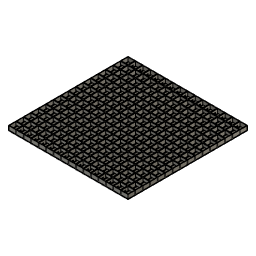
v0_base (Autodesk Fusion 360 design; units mm, degrees)
Autodesk Fusion 360 part; units mm, degrees
(part 1 of 2)
sketch "Skizze5" plane through (0, 0, 0) normal (0, 0, 1) x (1, 0, 0)
  line L0 (0, 272) -> (272, 272)
  line L1 (272, 272) -> (272, 0)
  line L2 (272, 0) -> (0, 0)
  line L3 (0, 0) -> (0, 272)
  dimension "d37" = 272
  dimension "d38" = 272
  constraint horizontal L0
  constraint vertical L1
  constraint horizontal L2
  constraint vertical L3
  constraint coincident L2.end L3.start
  measures "d37" distance of L0.start L0.end
  measures "d38" distance of L0.end L1.end
extrude "Extrusion4" add sketch "Skizze5" along normal blind 10
sketch "Skizze7" plane through (0, 0, 0) normal (0, 0, 1) x (1, 0, 0)
  line L0 (1, 16, 0.0025) -> (16, 16, 0.0025)
  line L1 (16, 16, 0.0025) -> (16, 1, 0.0025)
  line L2 (16, 1, 0.0025) -> (1, 1, 0.0025)
  line L3 (1, 1, 0.0025) -> (1, 16, 0.0025)
  line L4 (18, 16, 0.0025) -> (33, 16, 0.0025)
  line L5 (18, 1, 0.0025) -> (18, 16, 0.0025)
  line L6 (33, 16, 0.0025) -> (33, 1, 0.0025)
  line L7 (33, 1, 0.0025) -> (18, 1, 0.0025)
  line L8 (35, 16, 0.0025) -> (50, 16, 0.0025)
  line L9 (35, 1, 0.0025) -> (35, 16, 0.0025)
  line L10 (50, 16, 0.0025) -> (50, 1, 0.0025)
  line L11 (50, 1, 0.0025) -> (35, 1, 0.0025)
  line L12 (52, 16, 0.0025) -> (67, 16, 0.0025)
  line L13 (52, 1, 0.0025) -> (52, 16, 0.0025)
  line L14 (67, 16, 0.0025) -> (67, 1, 0.0025)
  line L15 (67, 1, 0.0025) -> (52, 1, 0.0025)
  line L16 (69, 16, 0.0025) -> (84, 16, 0.0025)
  line L17 (69, 1, 0.0025) -> (69, 16, 0.0025)
  line L18 (84, 16, 0.0025) -> (84, 1, 0.0025)
  line L19 (84, 1, 0.0025) -> (69, 1, 0.0025)
  line L20 (86, 16, 0.0025) -> (101, 16, 0.0025)
  line L21 (86, 1, 0.0025) -> (86, 16, 0.0025)
  line L22 (101, 16, 0.0025) -> (101, 1, 0.0025)
  line L23 (101, 1, 0.0025) -> (86, 1, 0.0025)
  line L24 (103, 16, 0.0025) -> (118, 16, 0.0025)
  line L25 (103, 1, 0.0025) -> (103, 16, 0.0025)
  line L26 (118, 16, 0.0025) -> (118, 1, 0.0025)
  line L27 (118, 1, 0.0025) -> (103, 1, 0.0025)
  line L28 (120, 16, 0.0025) -> (135, 16, 0.0025)
  line L29 (120, 1, 0.0025) -> (120, 16, 0.0025)
  line L30 (135, 16, 0.0025) -> (135, 1, 0.0025)
  line L31 (135, 1, 0.0025) -> (120, 1, 0.0025)
  line L32 (137, 16, 0.0025) -> (152, 16, 0.0025)
  line L33 (137, 1, 0.0025) -> (137, 16, 0.0025)
  line L34 (152, 16, 0.0025) -> (152, 1, 0.0025)
  line L35 (152, 1, 0.0025) -> (137, 1, 0.0025)
  line L36 (154, 16, 0.0025) -> (169, 16, 0.0025)
  line L37 (154, 1, 0.0025) -> (154, 16, 0.0025)
  line L38 (169, 16, 0.0025) -> (169, 1, 0.0025)
  line L39 (169, 1, 0.0025) -> (154, 1, 0.0025)
  line L40 (171, 16, 0.0025) -> (186, 16, 0.0025)
  line L41 (171, 1, 0.0025) -> (171, 16, 0.0025)
  line L42 (186, 16, 0.0025) -> (186, 1, 0.0025)
  line L43 (186, 1, 0.0025) -> (171, 1, 0.0025)
  line L44 (188, 16, 0.0025) -> (203, 16, 0.0025)
  line L45 (188, 1, 0.0025) -> (188, 16, 0.0025)
  line L46 (203, 16, 0.0025) -> (203, 1, 0.0025)
  line L47 (203, 1, 0.0025) -> (188, 1, 0.0025)
  line L48 (205, 16, 0.0025) -> (220, 16, 0.0025)
  line L49 (205, 1, 0.0025) -> (205, 16, 0.0025)
  line L50 (220, 16, 0.0025) -> (220, 1, 0.0025)
  line L51 (220, 1, 0.0025) -> (205, 1, 0.0025)
  line L52 (222, 16, 0.0025) -> (237, 16, 0.0025)
  line L53 (222, 1, 0.0025) -> (222, 16, 0.0025)
  line L54 (237, 16, 0.0025) -> (237, 1, 0.0025)
  line L55 (237, 1, 0.0025) -> (222, 1, 0.0025)
  line L56 (239, 16, 0.0025) -> (254, 16, 0.0025)
  line L57 (239, 1, 0.0025) -> (239, 16, 0.0025)
  line L58 (254, 16, 0.0025) -> (254, 1, 0.0025)
  line L59 (254, 1, 0.0025) -> (239, 1, 0.0025)
  line L60 (256, 16, 0.0025) -> (271, 16, 0.0025)
  line L61 (256, 1, 0.0025) -> (256, 16, 0.0025)
  line L62 (271, 16, 0.0025) -> (271, 1, 0.0025)
  line L63 (271, 1, 0.0025) -> (256, 1, 0.0025)
  line L64 (1, 33, 0.0025) -> (16, 33, 0.0025)
  line L65 (1, 18, 0.0025) -> (1, 33, 0.0025)
  line L66 (16, 33, 0.0025) -> (16, 18, 0.0025)
  line L67 (16, 18, 0.0025) -> (1, 18, 0.0025)
  line L68 (18, 33, 0.0025) -> (33, 33, 0.0025)
  line L69 (18, 18, 0.0025) -> (18, 33, 0.0025)
  line L70 (33, 33, 0.0025) -> (33, 18, 0.0025)
  line L71 (33, 18, 0.0025) -> (18, 18, 0.0025)
  line L72 (35, 33, 0.0025) -> (50, 33, 0.0025)
  line L73 (35, 18, 0.0025) -> (35, 33, 0.0025)
  line L74 (50, 33, 0.0025) -> (50, 18, 0.0025)
  line L75 (50, 18, 0.0025) -> (35, 18, 0.0025)
  line L76 (52, 33, 0.0025) -> (67, 33, 0.0025)
  line L77 (52, 18, 0.0025) -> (52, 33, 0.0025)
  line L78 (67, 33, 0.0025) -> (67, 18, 0.0025)
  line L79 (67, 18, 0.0025) -> (52, 18, 0.0025)
  line L80 (69, 33, 0.0025) -> (84, 33, 0.0025)
  line L81 (69, 18, 0.0025) -> (69, 33, 0.0025)
  line L82 (84, 33, 0.0025) -> (84, 18, 0.0025)
  line L83 (84, 18, 0.0025) -> (69, 18, 0.0025)
  line L84 (86, 33, 0.0025) -> (101, 33, 0.0025)
  line L85 (86, 18, 0.0025) -> (86, 33, 0.0025)
  line L86 (101, 33, 0.0025) -> (101, 18, 0.0025)
  line L87 (101, 18, 0.0025) -> (86, 18, 0.0025)
  line L88 (103, 33, 0.0025) -> (118, 33, 0.0025)
  line L89 (103, 18, 0.0025) -> (103, 33, 0.0025)
  line L90 (118, 33, 0.0025) -> (118, 18, 0.0025)
  line L91 (118, 18, 0.0025) -> (103, 18, 0.0025)
  line L92 (120, 33, 0.0025) -> (135, 33, 0.0025)
  line L93 (120, 18, 0.0025) -> (120, 33, 0.0025)
  line L94 (135, 33, 0.0025) -> (135, 18, 0.0025)
  line L95 (135, 18, 0.0025) -> (120, 18, 0.0025)
  line L96 (137, 33, 0.0025) -> (152, 33, 0.0025)
  line L97 (137, 18, 0.0025) -> (137, 33, 0.0025)
  line L98 (152, 33, 0.0025) -> (152, 18, 0.0025)
  line L99 (152, 18, 0.0025) -> (137, 18, 0.0025)
  line L100 (154, 33, 0.0025) -> (169, 33, 0.0025)
  line L101 (154, 18, 0.0025) -> (154, 33, 0.0025)
  line L102 (169, 33, 0.0025) -> (169, 18, 0.0025)
  line L103 (169, 18, 0.0025) -> (154, 18, 0.0025)
  line L104 (171, 33, 0.0025) -> (186, 33, 0.0025)
  line L105 (171, 18, 0.0025) -> (171, 33, 0.0025)
  line L106 (186, 33, 0.0025) -> (186, 18, 0.0025)
  line L107 (186, 18, 0.0025) -> (171, 18, 0.0025)
  line L108 (188, 33, 0.0025) -> (203, 33, 0.0025)
  line L109 (188, 18, 0.0025) -> (188, 33, 0.0025)
  line L110 (203, 33, 0.0025) -> (203, 18, 0.0025)
  line L111 (203, 18, 0.0025) -> (188, 18, 0.0025)
  line L112 (205, 33, 0.0025) -> (220, 33, 0.0025)
  line L113 (205, 18, 0.0025) -> (205, 33, 0.0025)
  line L114 (220, 33, 0.0025) -> (220, 18, 0.0025)
  line L115 (220, 18, 0.0025) -> (205, 18, 0.0025)
  line L116 (222, 33, 0.0025) -> (237, 33, 0.0025)
  line L117 (222, 18, 0.0025) -> (222, 33, 0.0025)
  line L118 (237, 33, 0.0025) -> (237, 18, 0.0025)
  line L119 (237, 18, 0.0025) -> (222, 18, 0.0025)
  line L120 (239, 33, 0.0025) -> (254, 33, 0.0025)
  line L121 (239, 18, 0.0025) -> (239, 33, 0.0025)
  line L122 (254, 33, 0.0025) -> (254, 18, 0.0025)
  line L123 (254, 18, 0.0025) -> (239, 18, 0.0025)
  line L124 (256, 33, 0.0025) -> (271, 33, 0.0025)
  line L125 (256, 18, 0.0025) -> (256, 33, 0.0025)
  line L126 (271, 33, 0.0025) -> (271, 18, 0.0025)
  line L127 (271, 18, 0.0025) -> (256, 18, 0.0025)
  line L128 (1, 50, 0.0025) -> (16, 50, 0.0025)
  line L129 (1, 35, 0.0025) -> (1, 50, 0.0025)
  line L130 (16, 50, 0.0025) -> (16, 35, 0.0025)
  line L131 (16, 35, 0.0025) -> (1, 35, 0.0025)
  line L132 (18, 50, 0.0025) -> (33, 50, 0.0025)
  line L133 (18, 35, 0.0025) -> (18, 50, 0.0025)
  line L134 (33, 50, 0.0025) -> (33, 35, 0.0025)
  line L135 (33, 35, 0.0025) -> (18, 35, 0.0025)
  line L136 (35, 50, 0.0025) -> (50, 50, 0.0025)
  line L137 (35, 35, 0.0025) -> (35, 50, 0.0025)
  line L138 (50, 50, 0.0025) -> (50, 35, 0.0025)
  line L139 (50, 35, 0.0025) -> (35, 35, 0.0025)
  line L140 (52, 50, 0.0025) -> (67, 50, 0.0025)
  line L141 (52, 35, 0.0025) -> (52, 50, 0.0025)
  line L142 (67, 50, 0.0025) -> (67, 35, 0.0025)
  line L143 (67, 35, 0.0025) -> (52, 35, 0.0025)
  line L144 (69, 50, 0.0025) -> (84, 50, 0.0025)
  line L145 (69, 35, 0.0025) -> (69, 50, 0.0025)
  line L146 (84, 50, 0.0025) -> (84, 35, 0.0025)
  line L147 (84, 35, 0.0025) -> (69, 35, 0.0025)
  line L148 (86, 50, 0.0025) -> (101, 50, 0.0025)
  line L149 (86, 35, 0.0025) -> (86, 50, 0.0025)
  line L150 (101, 50, 0.0025) -> (101, 35, 0.0025)
  line L151 (101, 35, 0.0025) -> (86, 35, 0.0025)
  line L152 (103, 50, 0.0025) -> (118, 50, 0.0025)
  line L153 (103, 35, 0.0025) -> (103, 50, 0.0025)
  line L154 (118, 50, 0.0025) -> (118, 35, 0.0025)
  line L155 (118, 35, 0.0025) -> (103, 35, 0.0025)
  line L156 (120, 50, 0.0025) -> (135, 50, 0.0025)
  line L157 (120, 35, 0.0025) -> (120, 50, 0.0025)
  line L158 (135, 50, 0.0025) -> (135, 35, 0.0025)
  line L159 (135, 35, 0.0025) -> (120, 35, 0.0025)
  line L160 (137, 50, 0.0025) -> (152, 50, 0.0025)
  line L161 (137, 35, 0.0025) -> (137, 50, 0.0025)
  line L162 (152, 50, 0.0025) -> (152, 35, 0.0025)
  line L163 (152, 35, 0.0025) -> (137, 35, 0.0025)
  line L164 (154, 50, 0.0025) -> (169, 50, 0.0025)
  line L165 (154, 35, 0.0025) -> (154, 50, 0.0025)
  line L166 (169, 50, 0.0025) -> (169, 35, 0.0025)
  line L167 (169, 35, 0.0025) -> (154, 35, 0.0025)
  line L168 (171, 50, 0.0025) -> (186, 50, 0.0025)
  line L169 (171, 35, 0.0025) -> (171, 50, 0.0025)
  line L170 (186, 50, 0.0025) -> (186, 35, 0.0025)
  line L171 (186, 35, 0.0025) -> (171, 35, 0.0025)
  line L172 (188, 50, 0.0025) -> (203, 50, 0.0025)
  line L173 (188, 35, 0.0025) -> (188, 50, 0.0025)
  line L174 (203, 50, 0.0025) -> (203, 35, 0.0025)
  line L175 (203, 35, 0.0025) -> (188, 35, 0.0025)
  line L176 (205, 50, 0.0025) -> (220, 50, 0.0025)
  line L177 (205, 35, 0.0025) -> (205, 50, 0.0025)
  line L178 (220, 50, 0.0025) -> (220, 35, 0.0025)
  line L179 (220, 35, 0.0025) -> (205, 35, 0.0025)
  line L180 (222, 50, 0.0025) -> (237, 50, 0.0025)
  line L181 (222, 35, 0.0025) -> (222, 50, 0.0025)
  line L182 (237, 50, 0.0025) -> (237, 35, 0.0025)
  line L183 (237, 35, 0.0025) -> (222, 35, 0.0025)
  line L184 (239, 50, 0.0025) -> (254, 50, 0.0025)
  line L185 (239, 35, 0.0025) -> (239, 50, 0.0025)
  line L186 (254, 50, 0.0025) -> (254, 35, 0.0025)
  line L187 (254, 35, 0.0025) -> (239, 35, 0.0025)
  line L188 (256, 50, 0.0025) -> (271, 50, 0.0025)
  line L189 (256, 35, 0.0025) -> (256, 50, 0.0025)
  line L190 (271, 50, 0.0025) -> (271, 35, 0.0025)
  line L191 (271, 35, 0.0025) -> (256, 35, 0.0025)
  line L192 (1, 67, 0.0025) -> (16, 67, 0.0025)
  line L193 (1, 52, 0.0025) -> (1, 67, 0.0025)
  line L194 (16, 67, 0.0025) -> (16, 52, 0.0025)
  line L195 (16, 52, 0.0025) -> (1, 52, 0.0025)
  line L196 (18, 67, 0.0025) -> (33, 67, 0.0025)
  line L197 (18, 52, 0.0025) -> (18, 67, 0.0025)
  line L198 (33, 67, 0.0025) -> (33, 52, 0.0025)
  line L199 (33, 52, 0.0025) -> (18, 52, 0.0025)
  line L200 (35, 67, 0.0025) -> (50, 67, 0.0025)
  line L201 (35, 52, 0.0025) -> (35, 67, 0.0025)
  line L202 (50, 67, 0.0025) -> (50, 52, 0.0025)
  line L203 (50, 52, 0.0025) -> (35, 52, 0.0025)
  line L204 (52, 67, 0.0025) -> (67, 67, 0.0025)
  line L205 (52, 52, 0.0025) -> (52, 67, 0.0025)
  line L206 (67, 67, 0.0025) -> (67, 52, 0.0025)
  line L207 (67, 52, 0.0025) -> (52, 52, 0.0025)
  line L208 (69, 67, 0.0025) -> (84, 67, 0.0025)
  line L209 (69, 52, 0.0025) -> (69, 67, 0.0025)
  line L210 (84, 67, 0.0025) -> (84, 52, 0.0025)
  line L211 (84, 52, 0.0025) -> (69, 52, 0.0025)
  line L212 (86, 67, 0.0025) -> (101, 67, 0.0025)
  line L213 (86, 52, 0.0025) -> (86, 67, 0.0025)
  line L214 (101, 67, 0.0025) -> (101, 52, 0.0025)
  line L215 (101, 52, 0.0025) -> (86, 52, 0.0025)
  line L216 (103, 67, 0.0025) -> (118, 67, 0.0025)
  line L217 (103, 52, 0.0025) -> (103, 67, 0.0025)
  line L218 (118, 67, 0.0025) -> (118, 52, 0.0025)
  line L219 (118, 52, 0.0025) -> (103, 52, 0.0025)
  line L220 (120, 67, 0.0025) -> (135, 67, 0.0025)
  line L221 (120, 52, 0.0025) -> (120, 67, 0.0025)
  line L222 (135, 67, 0.0025) -> (135, 52, 0.0025)
  line L223 (135, 52, 0.0025) -> (120, 52, 0.0025)
  line L224 (137, 67, 0.0025) -> (152, 67, 0.0025)
  line L225 (137, 52, 0.0025) -> (137, 67, 0.0025)
  line L226 (152, 67, 0.0025) -> (152, 52, 0.0025)
  line L227 (152, 52, 0.0025) -> (137, 52, 0.0025)
  line L228 (154, 67, 0.0025) -> (169, 67, 0.0025)
  line L229 (154, 52, 0.0025) -> (154, 67, 0.0025)
  line L230 (169, 67, 0.0025) -> (169, 52, 0.0025)
  line L231 (169, 52, 0.0025) -> (154, 52, 0.0025)
  line L232 (171, 67, 0.0025) -> (186, 67, 0.0025)
  line L233 (171, 52, 0.0025) -> (171, 67, 0.0025)
  line L234 (186, 67, 0.0025) -> (186, 52, 0.0025)
  line L235 (186, 52, 0.0025) -> (171, 52, 0.0025)
  line L236 (188, 67, 0.0025) -> (203, 67, 0.0025)
  line L237 (188, 52, 0.0025) -> (188, 67, 0.0025)
  line L238 (203, 67, 0.0025) -> (203, 52, 0.0025)
  line L239 (203, 52, 0.0025) -> (188, 52, 0.0025)
  line L240 (205, 67, 0.0025) -> (220, 67, 0.0025)
  line L241 (205, 52, 0.0025) -> (205, 67, 0.0025)
  line L242 (220, 67, 0.0025) -> (220, 52, 0.0025)
  line L243 (220, 52, 0.0025) -> (205, 52, 0.0025)
  line L244 (222, 67, 0.0025) -> (237, 67, 0.0025)
  line L245 (222, 52, 0.0025) -> (222, 67, 0.0025)
  line L246 (237, 67, 0.0025) -> (237, 52, 0.0025)
  line L247 (237, 52, 0.0025) -> (222, 52, 0.0025)
  line L248 (239, 67, 0.0025) -> (254, 67, 0.0025)
  line L249 (239, 52, 0.0025) -> (239, 67, 0.0025)
  line L250 (254, 67, 0.0025) -> (254, 52, 0.0025)
  line L251 (254, 52, 0.0025) -> (239, 52, 0.0025)
  line L252 (256, 67, 0.0025) -> (271, 67, 0.0025)
  line L253 (256, 52, 0.0025) -> (256, 67, 0.0025)
  line L254 (271, 67, 0.0025) -> (271, 52, 0.0025)
  line L255 (271, 52, 0.0025) -> (256, 52, 0.0025)
  line L256 (1, 84, 0.0025) -> (16, 84, 0.0025)
  line L257 (1, 69, 0.0025) -> (1, 84, 0.0025)
  line L258 (16, 84, 0.0025) -> (16, 69, 0.0025)
  line L259 (16, 69, 0.0025) -> (1, 69, 0.0025)
  line L260 (18, 84, 0.0025) -> (33, 84, 0.0025)
  line L261 (18, 69, 0.0025) -> (18, 84, 0.0025)
  line L262 (33, 84, 0.0025) -> (33, 69, 0.0025)
  line L263 (33, 69, 0.0025) -> (18, 69, 0.0025)
  line L264 (35, 84, 0.0025) -> (50, 84, 0.0025)
  line L265 (35, 69, 0.0025) -> (35, 84, 0.0025)
  line L266 (50, 84, 0.0025) -> (50, 69, 0.0025)
  line L267 (50, 69, 0.0025) -> (35, 69, 0.0025)
  line L268 (52, 84, 0.0025) -> (67, 84, 0.0025)
  line L269 (52, 69, 0.0025) -> (52, 84, 0.0025)
  line L270 (67, 84, 0.0025) -> (67, 69, 0.0025)
  line L271 (67, 69, 0.0025) -> (52, 69, 0.0025)
  line L272 (69, 84, 0.0025) -> (84, 84, 0.0025)
  line L273 (69, 69, 0.0025) -> (69, 84, 0.0025)
  line L274 (84, 84, 0.0025) -> (84, 69, 0.0025)
  line L275 (84, 69, 0.0025) -> (69, 69, 0.0025)
  line L276 (86, 84, 0.0025) -> (101, 84, 0.0025)
  line L277 (86, 69, 0.0025) -> (86, 84, 0.0025)
  line L278 (101, 84, 0.0025) -> (101, 69, 0.0025)
  line L279 (101, 69, 0.0025) -> (86, 69, 0.0025)
  line L280 (103, 84, 0.0025) -> (118, 84, 0.0025)
  line L281 (103, 69, 0.0025) -> (103, 84, 0.0025)
  line L282 (118, 84, 0.0025) -> (118, 69, 0.0025)
  line L283 (118, 69, 0.0025) -> (103, 69, 0.0025)
  line L284 (120, 84, 0.0025) -> (135, 84, 0.0025)
  line L285 (120, 69, 0.0025) -> (120, 84, 0.0025)
  line L286 (135, 84, 0.0025) -> (135, 69, 0.0025)
  line L287 (135, 69, 0.0025) -> (120, 69, 0.0025)
  line L288 (137, 84, 0.0025) -> (152, 84, 0.0025)
  line L289 (137, 69, 0.0025) -> (137, 84, 0.0025)
  line L290 (152, 84, 0.0025) -> (152, 69, 0.0025)
  line L291 (152, 69, 0.0025) -> (137, 69, 0.0025)
  line L292 (154, 84, 0.0025) -> (169, 84, 0.0025)
  line L293 (154, 69, 0.0025) -> (154, 84, 0.0025)
  line L294 (169, 84, 0.0025) -> (169, 69, 0.0025)
  line L295 (169, 69, 0.0025) -> (154, 69, 0.0025)
  line L296 (171, 84, 0.0025) -> (186, 84, 0.0025)
  line L297 (171, 69, 0.0025) -> (171, 84, 0.0025)
  line L298 (186, 84, 0.0025) -> (186, 69, 0.0025)
  line L299 (186, 69, 0.0025) -> (171, 69, 0.0025)
  line L300 (188, 84, 0.0025) -> (203, 84, 0.0025)
  line L301 (188, 69, 0.0025) -> (188, 84, 0.0025)
  line L302 (203, 84, 0.0025) -> (203, 69, 0.0025)
  line L303 (203, 69, 0.0025) -> (188, 69, 0.0025)
  line L304 (205, 84, 0.0025) -> (220, 84, 0.0025)
  line L305 (205, 69, 0.0025) -> (205, 84, 0.0025)
  line L306 (220, 84, 0.0025) -> (220, 69, 0.0025)
  line L307 (220, 69, 0.0025) -> (205, 69, 0.0025)
  line L308 (222, 84, 0.0025) -> (237, 84, 0.0025)
  line L309 (222, 69, 0.0025) -> (222, 84, 0.0025)
  line L310 (237, 84, 0.0025) -> (237, 69, 0.0025)
  line L311 (237, 69, 0.0025) -> (222, 69, 0.0025)
  line L312 (239, 84, 0.0025) -> (254, 84, 0.0025)
  line L313 (239, 69, 0.0025) -> (239, 84, 0.0025)
  line L314 (254, 84, 0.0025) -> (254, 69, 0.0025)
  line L315 (254, 69, 0.0025) -> (239, 69, 0.0025)
  line L316 (256, 84, 0.0025) -> (271, 84, 0.0025)
  line L317 (256, 69, 0.0025) -> (256, 84, 0.0025)
  line L318 (271, 84, 0.0025) -> (271, 69, 0.0025)
  line L319 (271, 69, 0.0025) -> (256, 69, 0.0025)
  line L320 (1, 101, 0.0025) -> (16, 101, 0.0025)
  line L321 (1, 86, 0.0025) -> (1, 101, 0.0025)
  line L322 (16, 101, 0.0025) -> (16, 86, 0.0025)
  line L323 (16, 86, 0.0025) -> (1, 86, 0.0025)
  line L324 (18, 101, 0.0025) -> (33, 101, 0.0025)
  line L325 (18, 86, 0.0025) -> (18, 101, 0.0025)
  line L326 (33, 101, 0.0025) -> (33, 86, 0.0025)
  line L327 (33, 86, 0.0025) -> (18, 86, 0.0025)
  line L328 (35, 101, 0.0025) -> (50, 101, 0.0025)
  line L329 (35, 86, 0.0025) -> (35, 101, 0.0025)
  line L330 (50, 101, 0.0025) -> (50, 86, 0.0025)
  line L331 (50, 86, 0.0025) -> (35, 86, 0.0025)
  line L332 (52, 101, 0.0025) -> (67, 101, 0.0025)
  line L333 (52, 86, 0.0025) -> (52, 101, 0.0025)
  line L334 (67, 101, 0.0025) -> (67, 86, 0.0025)
  line L335 (67, 86, 0.0025) -> (52, 86, 0.0025)
  line L336 (69, 101, 0.0025) -> (84, 101, 0.0025)
  line L337 (69, 86, 0.0025) -> (69, 101, 0.0025)
  line L338 (84, 101, 0.0025) -> (84, 86, 0.0025)
  line L339 (84, 86, 0.0025) -> (69, 86, 0.0025)
  line L340 (86, 101, 0.0025) -> (101, 101, 0.0025)
  line L341 (86, 86, 0.0025) -> (86, 101, 0.0025)
  line L342 (101, 101, 0.0025) -> (101, 86, 0.0025)
  line L343 (101, 86, 0.0025) -> (86, 86, 0.0025)
  line L344 (103, 101, 0.0025) -> (118, 101, 0.0025)
  line L345 (103, 86, 0.0025) -> (103, 101, 0.0025)
  line L346 (118, 101, 0.0025) -> (118, 86, 0.0025)
  line L347 (118, 86, 0.0025) -> (103, 86, 0.0025)
  line L348 (120, 101, 0.0025) -> (135, 101, 0.0025)
  line L349 (120, 86, 0.0025) -> (120, 101, 0.0025)
  line L350 (135, 101, 0.0025) -> (135, 86, 0.0025)
  line L351 (135, 86, 0.0025) -> (120, 86, 0.0025)
  line L352 (137, 101, 0.0025) -> (152, 101, 0.0025)
  line L353 (137, 86, 0.0025) -> (137, 101, 0.0025)
  line L354 (152, 101, 0.0025) -> (152, 86, 0.0025)
  line L355 (152, 86, 0.0025) -> (137, 86, 0.0025)
  line L356 (154, 101, 0.0025) -> (169, 101, 0.0025)
  line L357 (154, 86, 0.0025) -> (154, 101, 0.0025)
  line L358 (169, 101, 0.0025) -> (169, 86, 0.0025)
  line L359 (169, 86, 0.0025) -> (154, 86, 0.0025)
  line L360 (171, 101, 0.0025) -> (186, 101, 0.0025)
  line L361 (171, 86, 0.0025) -> (171, 101, 0.0025)
  line L362 (186, 101, 0.0025) -> (186, 86, 0.0025)
  line L363 (186, 86, 0.0025) -> (171, 86, 0.0025)
  line L364 (188, 101, 0.0025) -> (203, 101, 0.0025)
  line L365 (188, 86, 0.0025) -> (188, 101, 0.0025)
  line L366 (203, 101, 0.0025) -> (203, 86, 0.0025)
  line L367 (203, 86, 0.0025) -> (188, 86, 0.0025)
  line L368 (205, 101, 0.0025) -> (220, 101, 0.0025)
  line L369 (205, 86, 0.0025) -> (205, 101, 0.0025)
  line L370 (220, 101, 0.0025) -> (220, 86, 0.0025)
  line L371 (220, 86, 0.0025) -> (205, 86, 0.0025)
  line L372 (222, 101, 0.0025) -> (237, 101, 0.0025)
  line L373 (222, 86, 0.0025) -> (222, 101, 0.0025)
  line L374 (237, 101, 0.0025) -> (237, 86, 0.0025)
  line L375 (237, 86, 0.0025) -> (222, 86, 0.0025)
  line L376 (239, 101, 0.0025) -> (254, 101, 0.0025)
  line L377 (239, 86, 0.0025) -> (239, 101, 0.0025)
  line L378 (254, 101, 0.0025) -> (254, 86, 0.0025)
  line L379 (254, 86, 0.0025) -> (239, 86, 0.0025)
  line L380 (256, 101, 0.0025) -> (271, 101, 0.0025)
  line L381 (256, 86, 0.0025) -> (256, 101, 0.0025)
  line L382 (271, 101, 0.0025) -> (271, 86, 0.0025)
  line L383 (271, 86, 0.0025) -> (256, 86, 0.0025)
  line L384 (1, 118, 0.0025) -> (16, 118, 0.0025)
  line L385 (1, 103, 0.0025) -> (1, 118, 0.0025)
  line L386 (16, 118, 0.0025) -> (16, 103, 0.0025)
  line L387 (16, 103, 0.0025) -> (1, 103, 0.0025)
  line L388 (18, 118, 0.0025) -> (33, 118, 0.0025)
  line L389 (18, 103, 0.0025) -> (18, 118, 0.0025)
  line L390 (33, 118, 0.0025) -> (33, 103, 0.0025)
  line L391 (33, 103, 0.0025) -> (18, 103, 0.0025)
  line L392 (35, 118, 0.0025) -> (50, 118, 0.0025)
  line L393 (35, 103, 0.0025) -> (35, 118, 0.0025)
  line L394 (50, 118, 0.0025) -> (50, 103, 0.0025)
  line L395 (50, 103, 0.0025) -> (35, 103, 0.0025)
  line L396 (52, 118, 0.0025) -> (67, 118, 0.0025)
  line L397 (52, 103, 0.0025) -> (52, 118, 0.0025)
  line L398 (67, 118, 0.0025) -> (67, 103, 0.0025)
  line L399 (67, 103, 0.0025) -> (52, 103, 0.0025)
  line L400 (69, 118, 0.0025) -> (84, 118, 0.0025)
  line L401 (69, 103, 0.0025) -> (69, 118, 0.0025)
  line L402 (84, 118, 0.0025) -> (84, 103, 0.0025)
  line L403 (84, 103, 0.0025) -> (69, 103, 0.0025)
  line L404 (86, 118, 0.0025) -> (101, 118, 0.0025)
  line L405 (86, 103, 0.0025) -> (86, 118, 0.0025)
  line L406 (101, 118, 0.0025) -> (101, 103, 0.0025)
  line L407 (101, 103, 0.0025) -> (86, 103, 0.0025)
  line L408 (103, 118, 0.0025) -> (118, 118, 0.0025)
  line L409 (103, 103, 0.0025) -> (103, 118, 0.0025)
  line L410 (118, 118, 0.0025) -> (118, 103, 0.0025)
  line L411 (118, 103, 0.0025) -> (103, 103, 0.0025)
  line L412 (120, 118, 0.0025) -> (135, 118, 0.0025)
  line L413 (120, 103, 0.0025) -> (120, 118, 0.0025)
  line L414 (135, 118, 0.0025) -> (135, 103, 0.0025)
  line L415 (135, 103, 0.0025) -> (120, 103, 0.0025)
  line L416 (137, 118, 0.0025) -> (152, 118, 0.0025)
  line L417 (137, 103, 0.0025) -> (137, 118, 0.0025)
  line L418 (152, 118, 0.0025) -> (152, 103, 0.0025)
  line L419 (152, 103, 0.0025) -> (137, 103, 0.0025)
  line L420 (154, 118, 0.0025) -> (169, 118, 0.0025)
  line L421 (154, 103, 0.0025) -> (154, 118, 0.0025)
  line L422 (169, 118, 0.0025) -> (169, 103, 0.0025)
  line L423 (169, 103, 0.0025) -> (154, 103, 0.0025)
  line L424 (171, 118, 0.0025) -> (186, 118, 0.0025)
  line L425 (171, 103, 0.0025) -> (171, 118, 0.0025)
  line L426 (186, 118, 0.0025) -> (186, 103, 0.0025)
  line L427 (186, 103, 0.0025) -> (171, 103, 0.0025)
  line L428 (188, 118, 0.0025) -> (203, 118, 0.0025)
  line L429 (188, 103, 0.0025) -> (188, 118, 0.0025)
  line L430 (203, 118, 0.0025) -> (203, 103, 0.0025)
  line L431 (203, 103, 0.0025) -> (188, 103, 0.0025)
  line L432 (205, 118, 0.0025) -> (220, 118, 0.0025)
  line L433 (205, 103, 0.0025) -> (205, 118, 0.0025)
  line L434 (220, 118, 0.0025) -> (220, 103, 0.0025)
  line L435 (220, 103, 0.0025) -> (205, 103, 0.0025)
  line L436 (222, 118, 0.0025) -> (237, 118, 0.0025)
  line L437 (222, 103, 0.0025) -> (222, 118, 0.0025)
  line L438 (237, 118, 0.0025) -> (237, 103, 0.0025)
  line L439 (237, 103, 0.0025) -> (222, 103, 0.0025)
  line L440 (239, 118, 0.0025) -> (254, 118, 0.0025)
  line L441 (239, 103, 0.0025) -> (239, 118, 0.0025)
  line L442 (254, 118, 0.0025) -> (254, 103, 0.0025)
  line L443 (254, 103, 0.0025) -> (239, 103, 0.0025)
  line L444 (256, 118, 0.0025) -> (271, 118, 0.0025)
  line L445 (256, 103, 0.0025) -> (256, 118, 0.0025)
  line L446 (271, 118, 0.0025) -> (271, 103, 0.0025)
  line L447 (271, 103, 0.0025) -> (256, 103, 0.0025)
  line L448 (1, 135, 0.0025) -> (16, 135, 0.0025)
  line L449 (1, 120, 0.0025) -> (1, 135, 0.0025)
  line L450 (16, 135, 0.0025) -> (16, 120, 0.0025)
  line L451 (16, 120, 0.0025) -> (1, 120, 0.0025)
  line L452 (18, 135, 0.0025) -> (33, 135, 0.0025)
  line L453 (18, 120, 0.0025) -> (18, 135, 0.0025)
  line L454 (33, 135, 0.0025) -> (33, 120, 0.0025)
  line L455 (33, 120, 0.0025) -> (18, 120, 0.0025)
  line L456 (35, 135, 0.0025) -> (50, 135, 0.0025)
  line L457 (35, 120, 0.0025) -> (35, 135, 0.0025)
  line L458 (50, 135, 0.0025) -> (50, 120, 0.0025)
  line L459 (50, 120, 0.0025) -> (35, 120, 0.0025)
  line L460 (52, 135, 0.0025) -> (67, 135, 0.0025)
  line L461 (52, 120, 0.0025) -> (52, 135, 0.0025)
  line L462 (67, 135, 0.0025) -> (67, 120, 0.0025)
  line L463 (67, 120, 0.0025) -> (52, 120, 0.0025)
  line L464 (69, 135, 0.0025) -> (84, 135, 0.0025)
  line L465 (69, 120, 0.0025) -> (69, 135, 0.0025)
  line L466 (84, 135, 0.0025) -> (84, 120, 0.0025)
  line L467 (84, 120, 0.0025) -> (69, 120, 0.0025)
  line L468 (86, 135, 0.0025) -> (101, 135, 0.0025)
  line L469 (86, 120, 0.0025) -> (86, 135, 0.0025)
  line L470 (101, 135, 0.0025) -> (101, 120, 0.0025)
  line L471 (101, 120, 0.0025) -> (86, 120, 0.0025)
  line L472 (103, 135, 0.0025) -> (118, 135, 0.0025)
  line L473 (103, 120, 0.0025) -> (103, 135, 0.0025)
  line L474 (118, 135, 0.0025) -> (118, 120, 0.0025)
  line L475 (118, 120, 0.0025) -> (103, 120, 0.0025)
  line L476 (120, 135, 0.0025) -> (135, 135, 0.0025)
  line L477 (120, 120, 0.0025) -> (120, 135, 0.0025)
  line L478 (135, 135, 0.0025) -> (135, 120, 0.0025)
  line L479 (135, 120, 0.0025) -> (120, 120, 0.0025)
  line L480 (137, 135, 0.0025) -> (152, 135, 0.0025)
  line L481 (137, 120, 0.0025) -> (137, 135, 0.0025)
  line L482 (152, 135, 0.0025) -> (152, 120, 0.0025)
  line L483 (152, 120, 0.0025) -> (137, 120, 0.0025)
  line L484 (154, 135, 0.0025) -> (169, 135, 0.0025)
  line L485 (154, 120, 0.0025) -> (154, 135, 0.0025)
  line L486 (169, 135, 0.0025) -> (169, 120, 0.0025)
  line L487 (169, 120, 0.0025) -> (154, 120, 0.0025)
  line L488 (171, 135, 0.0025) -> (186, 135, 0.0025)
  line L489 (171, 120, 0.0025) -> (171, 135, 0.0025)
  line L490 (186, 135, 0.0025) -> (186, 120, 0.0025)
  line L491 (186, 120, 0.0025) -> (171, 120, 0.0025)
  line L492 (188, 135, 0.0025) -> (203, 135, 0.0025)
  line L493 (188, 120, 0.0025) -> (188, 135, 0.0025)
  line L494 (203, 135, 0.0025) -> (203, 120, 0.0025)
  line L495 (203, 120, 0.0025) -> (188, 120, 0.0025)
  line L496 (205, 135, 0.0025) -> (220, 135, 0.0025)
  line L497 (205, 120, 0.0025) -> (205, 135, 0.0025)
  line L498 (220, 135, 0.0025) -> (220, 120, 0.0025)
  line L499 (220, 120, 0.0025) -> (205, 120, 0.0025)
  line L500 (222, 135, 0.0025) -> (237, 135, 0.0025)
  line L501 (222, 120, 0.0025) -> (222, 135, 0.0025)
  line L502 (237, 135, 0.0025) -> (237, 120, 0.0025)
  line L503 (237, 120, 0.0025) -> (222, 120, 0.0025)
  line L504 (239, 135, 0.0025) -> (254, 135, 0.0025)
  line L505 (239, 120, 0.0025) -> (239, 135, 0.0025)
  line L506 (254, 135, 0.0025) -> (254, 120, 0.0025)
  line L507 (254, 120, 0.0025) -> (239, 120, 0.0025)
  line L508 (256, 135, 0.0025) -> (271, 135, 0.0025)
  line L509 (256, 120, 0.0025) -> (256, 135, 0.0025)
  line L510 (271, 135, 0.0025) -> (271, 120, 0.0025)
  line L511 (271, 120, 0.0025) -> (256, 120, 0.0025)
  line L512 (1, 152, 0.0025) -> (16, 152, 0.0025)
  line L513 (1, 137, 0.0025) -> (1, 152, 0.0025)
  line L514 (16, 152, 0.0025) -> (16, 137, 0.0025)
  line L515 (16, 137, 0.0025) -> (1, 137, 0.0025)
  line L516 (18, 152, 0.0025) -> (33, 152, 0.0025)
  line L517 (18, 137, 0.0025) -> (18, 152, 0.0025)
  line L518 (33, 152, 0.0025) -> (33, 137, 0.0025)
  line L519 (33, 137, 0.0025) -> (18, 137, 0.0025)
  line L520 (35, 152, 0.0025) -> (50, 152, 0.0025)
  line L521 (35, 137, 0.0025) -> (35, 152, 0.0025)
  line L522 (50, 152, 0.0025) -> (50, 137, 0.0025)
  line L523 (50, 137, 0.0025) -> (35, 137, 0.0025)
  line L524 (52, 152, 0.0025) -> (67, 152, 0.0025)
  line L525 (52, 137, 0.0025) -> (52, 152, 0.0025)
  line L526 (67, 152, 0.0025) -> (67, 137, 0.0025)
  line L527 (67, 137, 0.0025) -> (52, 137, 0.0025)
  line L528 (69, 152, 0.0025) -> (84, 152, 0.0025)
  line L529 (69, 137, 0.0025) -> (69, 152, 0.0025)
  line L530 (84, 152, 0.0025) -> (84, 137, 0.0025)
  line L531 (84, 137, 0.0025) -> (69, 137, 0.0025)
  line L532 (86, 152, 0.0025) -> (101, 152, 0.0025)
  line L533 (86, 137, 0.0025) -> (86, 152, 0.0025)
  line L534 (101, 152, 0.0025) -> (101, 137, 0.0025)
  line L535 (101, 137, 0.0025) -> (86, 137, 0.0025)
  line L536 (103, 152, 0.0025) -> (118, 152, 0.0025)
  line L537 (103, 137, 0.0025) -> (103, 152, 0.0025)
  line L538 (118, 152, 0.0025) -> (118, 137, 0.0025)
  line L539 (118, 137, 0.0025) -> (103, 137, 0.0025)
  line L540 (120, 152, 0.0025) -> (135, 152, 0.0025)
  line L541 (120, 137, 0.0025) -> (120, 152, 0.0025)
  line L542 (135, 152, 0.0025) -> (135, 137, 0.0025)
  line L543 (135, 137, 0.0025) -> (120, 137, 0.0025)
  line L544 (137, 152, 0.0025) -> (152, 152, 0.0025)
  line L545 (137, 137, 0.0025) -> (137, 152, 0.0025)
  line L546 (152, 152, 0.0025) -> (152, 137, 0.0025)
  line L547 (152, 137, 0.0025) -> (137, 137, 0.0025)
  line L548 (154, 152, 0.0025) -> (169, 152, 0.0025)
  line L549 (154, 137, 0.0025) -> (154, 152, 0.0025)
  line L550 (169, 152, 0.0025) -> (169, 137, 0.0025)
  line L551 (169, 137, 0.0025) -> (154, 137, 0.0025)
  line L552 (171, 152, 0.0025) -> (186, 152, 0.0025)
  line L553 (171, 137, 0.0025) -> (171, 152, 0.0025)
  line L554 (186, 152, 0.0025) -> (186, 137, 0.0025)
  line L555 (186, 137, 0.0025) -> (171, 137, 0.0025)
  line L556 (188, 152, 0.0025) -> (203, 152, 0.0025)
  line L557 (188, 137, 0.0025) -> (188, 152, 0.0025)
  line L558 (203, 152, 0.0025) -> (203, 137, 0.0025)
  line L559 (203, 137, 0.0025) -> (188, 137, 0.0025)
  line L560 (205, 152, 0.0025) -> (220, 152, 0.0025)
  line L561 (205, 137, 0.0025) -> (205, 152, 0.0025)
  line L562 (220, 152, 0.0025) -> (220, 137, 0.0025)
  line L563 (220, 137, 0.0025) -> (205, 137, 0.0025)
  line L564 (222, 152, 0.0025) -> (237, 152, 0.0025)
  line L565 (222, 137, 0.0025) -> (222, 152, 0.0025)
  line L566 (237, 152, 0.0025) -> (237, 137, 0.0025)
  line L567 (237, 137, 0.0025) -> (222, 137, 0.0025)
  line L568 (239, 152, 0.0025) -> (254, 152, 0.0025)
  line L569 (239, 137, 0.0025) -> (239, 152, 0.0025)
  line L570 (254, 152, 0.0025) -> (254, 137, 0.0025)
  line L571 (254, 137, 0.0025) -> (239, 137, 0.0025)
  line L572 (256, 152, 0.0025) -> (271, 152, 0.0025)
  line L573 (256, 137, 0.0025) -> (256, 152, 0.0025)
  line L574 (271, 152, 0.0025) -> (271, 137, 0.0025)
  line L575 (271, 137, 0.0025) -> (256, 137, 0.0025)
  line L576 (1, 169, 0.0025) -> (16, 169, 0.0025)
  line L577 (1, 154, 0.0025) -> (1, 169, 0.0025)
  line L578 (16, 169, 0.0025) -> (16, 154, 0.0025)
  line L579 (16, 154, 0.0025) -> (1, 154, 0.0025)
  line L580 (18, 169, 0.0025) -> (33, 169, 0.0025)
  line L581 (18, 154, 0.0025) -> (18, 169, 0.0025)
  line L582 (33, 169, 0.0025) -> (33, 154, 0.0025)
  line L583 (33, 154, 0.0025) -> (18, 154, 0.0025)
  line L584 (35, 169, 0.0025) -> (50, 169, 0.0025)
  line L585 (35, 154, 0.0025) -> (35, 169, 0.0025)
  line L586 (50, 169, 0.0025) -> (50, 154, 0.0025)
  line L587 (50, 154, 0.0025) -> (35, 154, 0.0025)
  line L588 (52, 169, 0.0025) -> (67, 169, 0.0025)
  line L589 (52, 154, 0.0025) -> (52, 169, 0.0025)
  line L590 (67, 169, 0.0025) -> (67, 154, 0.0025)
  line L591 (67, 154, 0.0025) -> (52, 154, 0.0025)
  line L592 (69, 169, 0.0025) -> (84, 169, 0.0025)
  line L593 (69, 154, 0.0025) -> (69, 169, 0.0025)
  line L594 (84, 169, 0.0025) -> (84, 154, 0.0025)
  line L595 (84, 154, 0.0025) -> (69, 154, 0.0025)
  line L596 (86, 169, 0.0025) -> (101, 169, 0.0025)
  line L597 (86, 154, 0.0025) -> (86, 169, 0.0025)
  line L598 (101, 169, 0.0025) -> (101, 154, 0.0025)
  line L599 (101, 154, 0.0025) -> (86, 154, 0.0025)
  line L600 (103, 169, 0.0025) -> (118, 169, 0.0025)
  line L601 (103, 154, 0.0025) -> (103, 169, 0.0025)
  line L602 (118, 169, 0.0025) -> (118, 154, 0.0025)
  line L603 (118, 154, 0.0025) -> (103, 154, 0.0025)
  line L604 (120, 169, 0.0025) -> (135, 169, 0.0025)
  line L605 (120, 154, 0.0025) -> (120, 169, 0.0025)
  line L606 (135, 169, 0.0025) -> (135, 154, 0.0025)
  line L607 (135, 154, 0.0025) -> (120, 154, 0.0025)
  line L608 (137, 169, 0.0025) -> (152, 169, 0.0025)
  line L609 (137, 154, 0.0025) -> (137, 169, 0.0025)
  line L610 (152, 169, 0.0025) -> (152, 154, 0.0025)
  line L611 (152, 154, 0.0025) -> (137, 154, 0.0025)
  line L612 (154, 169, 0.0025) -> (169, 169, 0.0025)
  line L613 (154, 154, 0.0025) -> (154, 169, 0.0025)
  line L614 (169, 169, 0.0025) -> (169, 154, 0.0025)
  line L615 (169, 154, 0.0025) -> (154, 154, 0.0025)
  line L616 (171, 169, 0.0025) -> (186, 169, 0.0025)
  line L617 (171, 154, 0.0025) -> (171, 169, 0.0025)
  line L618 (186, 169, 0.0025) -> (186, 154, 0.0025)
  line L619 (186, 154, 0.0025) -> (171, 154, 0.0025)
  line L620 (188, 169, 0.0025) -> (203, 169, 0.0025)
  line L621 (188, 154, 0.0025) -> (188, 169, 0.0025)
  line L622 (203, 169, 0.0025) -> (203, 154, 0.0025)
  line L623 (203, 154, 0.0025) -> (188, 154, 0.0025)
  line L624 (205, 169, 0.0025) -> (220, 169, 0.0025)
  line L625 (205, 154, 0.0025) -> (205, 169, 0.0025)
  line L626 (220, 169, 0.0025) -> (220, 154, 0.0025)
  line L627 (220, 154, 0.0025) -> (205, 154, 0.0025)
  line L628 (222, 169, 0.0025) -> (237, 169, 0.0025)
  line L629 (222, 154, 0.0025) -> (222, 169, 0.0025)
  line L630 (237, 169, 0.0025) -> (237, 154, 0.0025)
  line L631 (237, 154, 0.0025) -> (222, 154, 0.0025)
  line L632 (239, 169, 0.0025) -> (254, 169, 0.0025)
  line L633 (239, 154, 0.0025) -> (239, 169, 0.0025)
  line L634 (254, 169, 0.0025) -> (254, 154, 0.0025)
  line L635 (254, 154, 0.0025) -> (239, 154, 0.0025)
  line L636 (256, 169, 0.0025) -> (271, 169, 0.0025)
  line L637 (256, 154, 0.0025) -> (256, 169, 0.0025)
  line L638 (271, 169, 0.0025) -> (271, 154, 0.0025)
  line L639 (271, 154, 0.0025) -> (256, 154, 0.0025)
  line L640 (1, 186, 0.0025) -> (16, 186, 0.0025)
  line L641 (1, 171, 0.0025) -> (1, 186, 0.0025)
  line L642 (16, 186, 0.0025) -> (16, 171, 0.0025)
  line L643 (16, 171, 0.0025) -> (1, 171, 0.0025)
  line L644 (18, 186, 0.0025) -> (33, 186, 0.0025)
  line L645 (18, 171, 0.0025) -> (18, 186, 0.0025)
  line L646 (33, 186, 0.0025) -> (33, 171, 0.0025)
  line L647 (33, 171, 0.0025) -> (18, 171, 0.0025)
  line L648 (35, 186, 0.0025) -> (50, 186, 0.0025)
  line L649 (35, 171, 0.0025) -> (35, 186, 0.0025)
  line L650 (50, 186, 0.0025) -> (50, 171, 0.0025)
  line L651 (50, 171, 0.0025) -> (35, 171, 0.0025)
  line L652 (52, 186, 0.0025) -> (67, 186, 0.0025)
  line L653 (52, 171, 0.0025) -> (52, 186, 0.0025)
  line L654 (67, 186, 0.0025) -> (67, 171, 0.0025)
  line L655 (67, 171, 0.0025) -> (52, 171, 0.0025)
  line L656 (69, 186, 0.0025) -> (84, 186, 0.0025)
  line L657 (69, 171, 0.0025) -> (69, 186, 0.0025)
  line L658 (84, 186, 0.0025) -> (84, 171, 0.0025)
  line L659 (84, 171, 0.0025) -> (69, 171, 0.0025)
  line L660 (86, 186, 0.0025) -> (101, 186, 0.0025)
  line L661 (86, 171, 0.0025) -> (86, 186, 0.0025)
  line L662 (101, 186, 0.0025) -> (101, 171, 0.0025)
  line L663 (101, 171, 0.0025) -> (86, 171, 0.0025)
  line L664 (103, 186, 0.0025) -> (118, 186, 0.0025)
  line L665 (103, 171, 0.0025) -> (103, 186, 0.0025)
  line L666 (118, 186, 0.0025) -> (118, 171, 0.0025)
  line L667 (118, 171, 0.0025) -> (103, 171, 0.0025)
  line L668 (120, 186, 0.0025) -> (135, 186, 0.0025)
  line L669 (120, 171, 0.0025) -> (120, 186, 0.0025)
  line L670 (135, 186, 0.0025) -> (135, 171, 0.0025)
  line L671 (135, 171, 0.0025) -> (120, 171, 0.0025)
  line L672 (137, 186, 0.0025) -> (152, 186, 0.0025)
  line L673 (137, 171, 0.0025) -> (137, 186, 0.0025)
  line L674 (152, 186, 0.0025) -> (152, 171, 0.0025)
  line L675 (152, 171, 0.0025) -> (137, 171, 0.0025)
  line L676 (154, 186, 0.0025) -> (169, 186, 0.0025)
  line L677 (154, 171, 0.0025) -> (154, 186, 0.0025)
  line L678 (169, 186, 0.0025) -> (169, 171, 0.0025)
  line L679 (169, 171, 0.0025) -> (154, 171, 0.0025)
  line L680 (171, 186, 0.0025) -> (186, 186, 0.0025)
  line L681 (171, 171, 0.0025) -> (171, 186, 0.0025)
  line L682 (186, 186, 0.0025) -> (186, 171, 0.0025)
  line L683 (186, 171, 0.0025) -> (171, 171, 0.0025)
  line L684 (188, 186, 0.0025) -> (203, 186, 0.0025)
  line L685 (188, 171, 0.0025) -> (188, 186, 0.0025)
  line L686 (203, 186, 0.0025) -> (203, 171, 0.0025)
  line L687 (203, 171, 0.0025) -> (188, 171, 0.0025)
  line L688 (205, 186, 0.0025) -> (220, 186, 0.0025)
  line L689 (205, 171, 0.0025) -> (205, 186, 0.0025)
  line L690 (220, 186, 0.0025) -> (220, 171, 0.0025)
  line L691 (220, 171, 0.0025) -> (205, 171, 0.0025)
  line L692 (222, 186, 0.0025) -> (237, 186, 0.0025)
  line L693 (222, 171, 0.0025) -> (222, 186, 0.0025)
  line L694 (237, 186, 0.0025) -> (237, 171, 0.0025)
  line L695 (237, 171, 0.0025) -> (222, 171, 0.0025)
  line L696 (239, 186, 0.0025) -> (254, 186, 0.0025)
  line L697 (239, 171, 0.0025) -> (239, 186, 0.0025)
  line L698 (254, 186, 0.0025) -> (254, 171, 0.0025)
  line L699 (254, 171, 0.0025) -> (239, 171, 0.0025)
  line L700 (256, 186, 0.0025) -> (271, 186, 0.0025)
  line L701 (256, 171, 0.0025) -> (256, 186, 0.0025)
  line L702 (271, 186, 0.0025) -> (271, 171, 0.0025)
  line L703 (271, 171, 0.0025) -> (256, 171, 0.0025)
  line L704 (1, 203, 0.0025) -> (16, 203, 0.0025)
  line L705 (1, 188, 0.0025) -> (1, 203, 0.0025)
  line L706 (16, 203, 0.0025) -> (16, 188, 0.0025)
  line L707 (16, 188, 0.0025) -> (1, 188, 0.0025)
  line L708 (18, 203, 0.0025) -> (33, 203, 0.0025)
  line L709 (18, 188, 0.0025) -> (18, 203, 0.0025)
  line L710 (33, 203, 0.0025) -> (33, 188, 0.0025)
  line L711 (33, 188, 0.0025) -> (18, 188, 0.0025)
  line L712 (35, 203, 0.0025) -> (50, 203, 0.0025)
  line L713 (35, 188, 0.0025) -> (35, 203, 0.0025)
  line L714 (50, 203, 0.0025) -> (50, 188, 0.0025)
  line L715 (50, 188, 0.0025) -> (35, 188, 0.0025)
  line L716 (52, 203, 0.0025) -> (67, 203, 0.0025)
  line L717 (52, 188, 0.0025) -> (52, 203, 0.0025)
  line L718 (67, 203, 0.0025) -> (67, 188, 0.0025)
  line L719 (67, 188, 0.0025) -> (52, 188, 0.0025)
  line L720 (69, 203, 0.0025) -> (84, 203, 0.0025)
  line L721 (69, 188, 0.0025) -> (69, 203, 0.0025)
  line L722 (84, 203, 0.0025) -> (84, 188, 0.0025)
  line L723 (84, 188, 0.0025) -> (69, 188, 0.0025)
  line L724 (86, 203, 0.0025) -> (101, 203, 0.0025)
  line L725 (86, 188, 0.0025) -> (86, 203, 0.0025)
  line L726 (101, 203, 0.0025) -> (101, 188, 0.0025)
  line L727 (101, 188, 0.0025) -> (86, 188, 0.0025)
  line L728 (103, 203, 0.0025) -> (118, 203, 0.0025)
  line L729 (103, 188, 0.0025) -> (103, 203, 0.0025)
  line L730 (118, 203, 0.0025) -> (118, 188, 0.0025)
  line L731 (118, 188, 0.0025) -> (103, 188, 0.0025)
  line L732 (120, 203, 0.0025) -> (135, 203, 0.0025)
  line L733 (120, 188, 0.0025) -> (120, 203, 0.0025)
  line L734 (135, 203, 0.0025) -> (135, 188, 0.0025)
  line L735 (135, 188, 0.0025) -> (120, 188, 0.0025)
  line L736 (137, 203, 0.0025) -> (152, 203, 0.0025)
  line L737 (137, 188, 0.0025) -> (137, 203, 0.0025)
  line L738 (152, 203, 0.0025) -> (152, 188, 0.0025)
  line L739 (152, 188, 0.0025) -> (137, 188, 0.0025)
  line L740 (154, 203, 0.0025) -> (169, 203, 0.0025)
  line L741 (154, 188, 0.0025) -> (154, 203, 0.0025)
  line L742 (169, 203, 0.0025) -> (169, 188, 0.0025)
  line L743 (169, 188, 0.0025) -> (154, 188, 0.0025)
  line L744 (171, 203, 0.0025) -> (186, 203, 0.0025)
  line L745 (171, 188, 0.0025) -> (171, 203, 0.0025)
  line L746 (186, 203, 0.0025) -> (186, 188, 0.0025)
  line L747 (186, 188, 0.0025) -> (171, 188, 0.0025)
  line L748 (188, 203, 0.0025) -> (203, 203, 0.0025)
  line L749 (188, 188, 0.0025) -> (188, 203, 0.0025)
  line L750 (203, 203, 0.0025) -> (203, 188, 0.0025)
  line L751 (203, 188, 0.0025) -> (188, 188, 0.0025)
  line L752 (205, 203, 0.0025) -> (220, 203, 0.0025)
  line L753 (205, 188, 0.0025) -> (205, 203, 0.0025)
  line L754 (220, 203, 0.0025) -> (220, 188, 0.0025)
  line L755 (220, 188, 0.0025) -> (205, 188, 0.0025)
  line L756 (222, 203, 0.0025) -> (237, 203, 0.0025)
  line L757 (222, 188, 0.0025) -> (222, 203, 0.0025)
  line L758 (237, 203, 0.0025) -> (237, 188, 0.0025)
  line L759 (237, 188, 0.0025) -> (222, 188, 0.0025)
  line L760 (239, 203, 0.0025) -> (254, 203, 0.0025)
  line L761 (239, 188, 0.0025) -> (239, 203, 0.0025)
  line L762 (254, 203, 0.0025) -> (254, 188, 0.0025)
  line L763 (254, 188, 0.0025) -> (239, 188, 0.0025)
  line L764 (256, 203, 0.0025) -> (271, 203, 0.0025)
  line L765 (256, 188, 0.0025) -> (256, 203, 0.0025)
  line L766 (271, 203, 0.0025) -> (271, 188, 0.0025)
  line L767 (271, 188, 0.0025) -> (256, 188, 0.0025)
  line L768 (1, 220, 0.0025) -> (16, 220, 0.0025)
  line L769 (1, 205, 0.0025) -> (1, 220, 0.0025)
  line L770 (16, 220, 0.0025) -> (16, 205, 0.0025)
  line L771 (16, 205, 0.0025) -> (1, 205, 0.0025)
  line L772 (18, 220, 0.0025) -> (33, 220, 0.0025)
  line L773 (18, 205, 0.0025) -> (18, 220, 0.0025)
  line L774 (33, 220, 0.0025) -> (33, 205, 0.0025)
  line L775 (33, 205, 0.0025) -> (18, 205, 0.0025)
  line L776 (35, 220, 0.0025) -> (50, 220, 0.0025)
  line L777 (35, 205, 0.0025) -> (35, 220, 0.0025)
  line L778 (50, 220, 0.0025) -> (50, 205, 0.0025)
  line L779 (50, 205, 0.0025) -> (35, 205, 0.0025)
  line L780 (52, 220, 0.0025) -> (67, 220, 0.0025)
  line L781 (52, 205, 0.0025) -> (52, 220, 0.0025)
  line L782 (67, 220, 0.0025) -> (67, 205, 0.0025)
  line L783 (67, 205, 0.0025) -> (52, 205, 0.0025)
  line L784 (69, 220, 0.0025) -> (84, 220, 0.0025)
  line L785 (69, 205, 0.0025) -> (69, 220, 0.0025)
  line L786 (84, 220, 0.0025) -> (84, 205, 0.0025)
  line L787 (84, 205, 0.0025) -> (69, 205, 0.0025)
  line L788 (86, 220, 0.0025) -> (101, 220, 0.0025)
  line L789 (86, 205, 0.0025) -> (86, 220, 0.0025)
  line L790 (101, 220, 0.0025) -> (101, 205, 0.0025)
  line L791 (101, 205, 0.0025) -> (86, 205, 0.0025)
  line L792 (103, 220, 0.0025) -> (118, 220, 0.0025)
  line L793 (103, 205, 0.0025) -> (103, 220, 0.0025)
  line L794 (118, 220, 0.0025) -> (118, 205, 0.0025)
  line L795 (118, 205, 0.0025) -> (103, 205, 0.0025)
  line L796 (120, 220, 0.0025) -> (135, 220, 0.0025)
  line L797 (120, 205, 0.0025) -> (120, 220, 0.0025)
  line L798 (135, 220, 0.0025) -> (135, 205, 0.0025)
  line L799 (135, 205, 0.0025) -> (120, 205, 0.0025)
  line L800 (137, 220, 0.0025) -> (152, 220, 0.0025)
  line L801 (137, 205, 0.0025) -> (137, 220, 0.0025)
  line L802 (152, 220, 0.0025) -> (152, 205, 0.0025)
  line L803 (152, 205, 0.0025) -> (137, 205, 0.0025)
  line L804 (154, 220, 0.0025) -> (169, 220, 0.0025)
  line L805 (154, 205, 0.0025) -> (154, 220, 0.0025)
  line L806 (169, 220, 0.0025) -> (169, 205, 0.0025)
  line L807 (169, 205, 0.0025) -> (154, 205, 0.0025)
  line L808 (171, 220, 0.0025) -> (186, 220, 0.0025)
  line L809 (171, 205, 0.0025) -> (171, 220, 0.0025)
  line L810 (186, 220, 0.0025) -> (186, 205, 0.0025)
  line L811 (186, 205, 0.0025) -> (171, 205, 0.0025)
  line L812 (188, 220, 0.0025) -> (203, 220, 0.0025)
  line L813 (188, 205, 0.0025) -> (188, 220, 0.0025)
  line L814 (203, 220, 0.0025) -> (203, 205, 0.0025)
  line L815 (203, 205, 0.0025) -> (188, 205, 0.0025)
  line L816 (205, 220, 0.0025) -> (220, 220, 0.0025)
  line L817 (205, 205, 0.0025) -> (205, 220, 0.0025)
  line L818 (220, 220, 0.0025) -> (220, 205, 0.0025)
  line L819 (220, 205, 0.0025) -> (205, 205, 0.0025)
  line L820 (222, 220, 0.0025) -> (237, 220, 0.0025)
  line L821 (222, 205, 0.0025) -> (222, 220, 0.0025)
  line L822 (237, 220, 0.0025) -> (237, 205, 0.0025)
  line L823 (237, 205, 0.0025) -> (222, 205, 0.0025)
  line L824 (239, 220, 0.0025) -> (254, 220, 0.0025)
  line L825 (239, 205, 0.0025) -> (239, 220, 0.0025)
  line L826 (254, 220, 0.0025) -> (254, 205, 0.0025)
  line L827 (254, 205, 0.0025) -> (239, 205, 0.0025)
  line L828 (256, 220, 0.0025) -> (271, 220, 0.0025)
  line L829 (256, 205, 0.0025) -> (256, 220, 0.0025)
  line L830 (271, 220, 0.0025) -> (271, 205, 0.0025)
  line L831 (271, 205, 0.0025) -> (256, 205, 0.0025)
  line L832 (1, 237, 0.0025) -> (16, 237, 0.0025)
  line L833 (1, 222, 0.0025) -> (1, 237, 0.0025)
  line L834 (16, 237, 0.0025) -> (16, 222, 0.0025)
  line L835 (16, 222, 0.0025) -> (1, 222, 0.0025)
  line L836 (18, 237, 0.0025) -> (33, 237, 0.0025)
  line L837 (18, 222, 0.0025) -> (18, 237, 0.0025)
  line L838 (33, 237, 0.0025) -> (33, 222, 0.0025)
  line L839 (33, 222, 0.0025) -> (18, 222, 0.0025)
  line L840 (35, 237, 0.0025) -> (50, 237, 0.0025)
  line L841 (35, 222, 0.0025) -> (35, 237, 0.0025)
  line L842 (50, 237, 0.0025) -> (50, 222, 0.0025)
  line L843 (50, 222, 0.0025) -> (35, 222, 0.0025)
  line L844 (52, 237, 0.0025) -> (67, 237, 0.0025)
  line L845 (52, 222, 0.0025) -> (52, 237, 0.0025)
  line L846 (67, 237, 0.0025) -> (67, 222, 0.0025)
  line L847 (67, 222, 0.0025) -> (52, 222, 0.0025)
  line L848 (69, 237, 0.0025) -> (84, 237, 0.0025)
  line L849 (69, 222, 0.0025) -> (69, 237, 0.0025)
  line L850 (84, 237, 0.0025) -> (84, 222, 0.0025)
  line L851 (84, 222, 0.0025) -> (69, 222, 0.0025)
  line L852 (86, 237, 0.0025) -> (101, 237, 0.0025)
  line L853 (86, 222, 0.0025) -> (86, 237, 0.0025)
  line L854 (101, 237, 0.0025) -> (101, 222, 0.0025)
  line L855 (101, 222, 0.0025) -> (86, 222, 0.0025)
  line L856 (103, 237, 0.0025) -> (118, 237, 0.0025)
  line L857 (103, 222, 0.0025) -> (103, 237, 0.0025)
  line L858 (118, 237, 0.0025) -> (118, 222, 0.0025)
  line L859 (118, 222, 0.0025) -> (103, 222, 0.0025)
  line L860 (120, 237, 0.0025) -> (135, 237, 0.0025)
  line L861 (120, 222, 0.0025) -> (120, 237, 0.0025)
  line L862 (135, 237, 0.0025) -> (135, 222, 0.0025)
  line L863 (135, 222, 0.0025) -> (120, 222, 0.0025)
  line L864 (137, 237, 0.0025) -> (152, 237, 0.0025)
  line L865 (137, 222, 0.0025) -> (137, 237, 0.0025)
  line L866 (152, 237, 0.0025) -> (152, 222, 0.0025)
  line L867 (152, 222, 0.0025) -> (137, 222, 0.0025)
  line L868 (154, 237, 0.0025) -> (169, 237, 0.0025)
  line L869 (154, 222, 0.0025) -> (154, 237, 0.0025)
  line L870 (169, 237, 0.0025) -> (169, 222, 0.0025)
  line L871 (169, 222, 0.0025) -> (154, 222, 0.0025)
  line L872 (171, 237, 0.0025) -> (186, 237, 0.0025)
  line L873 (171, 222, 0.0025) -> (171, 237, 0.0025)
  line L874 (186, 237, 0.0025) -> (186, 222, 0.0025)
  line L875 (186, 222, 0.0025) -> (171, 222, 0.0025)
  line L876 (188, 237, 0.0025) -> (203, 237, 0.0025)
  line L877 (188, 222, 0.0025) -> (188, 237, 0.0025)
  line L878 (203, 237, 0.0025) -> (203, 222, 0.0025)
  line L879 (203, 222, 0.0025) -> (188, 222, 0.0025)
  line L880 (205, 237, 0.0025) -> (220, 237, 0.0025)
  line L881 (205, 222, 0.0025) -> (205, 237, 0.0025)
  line L882 (220, 237, 0.0025) -> (220, 222, 0.0025)
  line L883 (220, 222, 0.0025) -> (205, 222, 0.0025)
  line L884 (222, 237, 0.0025) -> (237, 237, 0.0025)
  line L885 (222, 222, 0.0025) -> (222, 237, 0.0025)
  line L886 (237, 237, 0.0025) -> (237, 222, 0.0025)
  line L887 (237, 222, 0.0025) -> (222, 222, 0.0025)
  line L888 (239, 237, 0.0025) -> (254, 237, 0.0025)
  line L889 (239, 222, 0.0025) -> (239, 237, 0.0025)
  line L890 (254, 237, 0.0025) -> (254, 222, 0.0025)
  line L891 (254, 222, 0.0025) -> (239, 222, 0.0025)
  line L892 (256, 237, 0.0025) -> (271, 237, 0.0025)
  line L893 (256, 222, 0.0025) -> (256, 237, 0.0025)
  line L894 (271, 237, 0.0025) -> (271, 222, 0.0025)
  line L895 (271, 222, 0.0025) -> (256, 222, 0.0025)
  line L896 (1, 254, 0.0025) -> (16, 254, 0.0025)
  line L897 (1, 239, 0.0025) -> (1, 254, 0.0025)
  line L898 (16, 254, 0.0025) -> (16, 239, 0.0025)
  line L899 (16, 239, 0.0025) -> (1, 239, 0.0025)
  line L900 (18, 254, 0.0025) -> (33, 254, 0.0025)
  line L901 (18, 239, 0.0025) -> (18, 254, 0.0025)
  line L902 (33, 254, 0.0025) -> (33, 239, 0.0025)
  line L903 (33, 239, 0.0025) -> (18, 239, 0.0025)
  line L904 (35, 254, 0.0025) -> (50, 254, 0.0025)
  line L905 (35, 239, 0.0025) -> (35, 254, 0.0025)
  line L906 (50, 254, 0.0025) -> (50, 239, 0.0025)
  line L907 (50, 239, 0.0025) -> (35, 239, 0.0025)
  line L908 (52, 254, 0.0025) -> (67, 254, 0.0025)
  line L909 (52, 239, 0.0025) -> (52, 254, 0.0025)
  line L910 (67, 254, 0.0025) -> (67, 239, 0.0025)
  line L911 (67, 239, 0.0025) -> (52, 239, 0.0025)
  line L912 (69, 254, 0.0025) -> (84, 254, 0.0025)
  line L913 (69, 239, 0.0025) -> (69, 254, 0.0025)
  line L914 (84, 254, 0.0025) -> (84, 239, 0.0025)
  line L915 (84, 239, 0.0025) -> (69, 239, 0.0025)
  line L916 (86, 254, 0.0025) -> (101, 254, 0.0025)
  line L917 (86, 239, 0.0025) -> (86, 254, 0.0025)
  line L918 (101, 254, 0.0025) -> (101, 239, 0.0025)
  line L919 (101, 239, 0.0025) -> (86, 239, 0.0025)
  line L920 (103, 254, 0.0025) -> (118, 254, 0.0025)
  line L921 (103, 239, 0.0025) -> (103, 254, 0.0025)
  line L922 (118, 254, 0.0025) -> (118, 239, 0.0025)
  line L923 (118, 239, 0.0025) -> (103, 239, 0.0025)
  line L924 (120, 254, 0.0025) -> (135, 254, 0.0025)
  line L925 (120, 239, 0.0025) -> (120, 254, 0.0025)
  line L926 (135, 254, 0.0025) -> (135, 239, 0.0025)
  line L927 (135, 239, 0.0025) -> (120, 239, 0.0025)
  line L928 (137, 254, 0.0025) -> (152, 254, 0.0025)
  line L929 (137, 239, 0.0025) -> (137, 254, 0.0025)
  line L930 (152, 254, 0.0025) -> (152, 239, 0.0025)
  line L931 (152, 239, 0.0025) -> (137, 239, 0.0025)
  line L932 (154, 254, 0.0025) -> (169, 254, 0.0025)
  line L933 (154, 239, 0.0025) -> (154, 254, 0.0025)
  line L934 (169, 254, 0.0025) -> (169, 239, 0.0025)
  line L935 (169, 239, 0.0025) -> (154, 239, 0.0025)
  line L936 (171, 254, 0.0025) -> (186, 254, 0.0025)
  line L937 (171, 239, 0.0025) -> (171, 254, 0.0025)
  line L938 (186, 254, 0.0025) -> (186, 239, 0.0025)
  line L939 (186, 239, 0.0025) -> (171, 239, 0.0025)
  line L940 (188, 254, 0.0025) -> (203, 254, 0.0025)
  line L941 (188, 239, 0.0025) -> (188, 254, 0.0025)
  line L942 (203, 254, 0.0025) -> (203, 239, 0.0025)
  line L943 (203, 239, 0.0025) -> (188, 239, 0.0025)
  line L944 (205, 254, 0.0025) -> (220, 254, 0.0025)
  line L945 (205, 239, 0.0025) -> (205, 254, 0.0025)
  line L946 (220, 254, 0.0025) -> (220, 239, 0.0025)
  line L947 (220, 239, 0.0025) -> (205, 239, 0.0025)
  line L948 (222, 254, 0.0025) -> (237, 254, 0.0025)
  line L949 (222, 239, 0.0025) -> (222, 254, 0.0025)
  line L950 (237, 254, 0.0025) -> (237, 239, 0.0025)
  line L951 (237, 239, 0.0025) -> (222, 239, 0.0025)
  line L952 (239, 254, 0.0025) -> (254, 254, 0.0025)
  line L953 (239, 239, 0.0025) -> (239, 254, 0.0025)
  line L954 (254, 254, 0.0025) -> (254, 239, 0.0025)
  line L955 (254, 239, 0.0025) -> (239, 239, 0.0025)
  line L956 (256, 254, 0.0025) -> (271, 254, 0.0025)
  line L957 (256, 239, 0.0025) -> (256, 254, 0.0025)